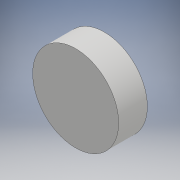
# Autodesk Inventor part: Spacer
Saved by Autodesk Inventor 2017 (Build 210142000, 142)
## iProperties
Created: 2018-02-08
Part Number: Spacer
Material: Generic
Document SubType Name: Modeling
Designer: Arjuna
Density: 1 g/cm^3
Appearance: Default
Author: Arjuna
Autodesk Inventor part; units mm, degrees
ref_plane "YZ Plane" through (0, 0, 0) normal (1, 0, 0) x (0, 1, 0)
ref_plane "XZ Plane" through (0, 0, 0) normal (0, 1, 0) x (-1, 0, 0)
ref_plane "XY Plane" through (0, 0, 0) normal (0, 0, 1) x (1, 0, 0)
sketch "Sketch1" plane through (0, 0, 0) normal (0, 0, 1) x (1, 0, 0)
  line L0 (0, 0) -> (7.5, 0)
  line L1 (7.5, 0) -> (7.5, 5)
  line L2 (7.5, 5) -> (0, 5)
  line L3 (0, 5) -> (0, 0)
  dimension "d0" = 7.5
  dimension "d1" = 5
  constraints: 8 end point, 2 horizontal, 2 perpendicular
  measures "d0" distance of L0.start L0.end
  measures "d1" distance of L0.end L1.end
revolve "Revolution1" add sketch "Sketch1" angle 360 about axis through (0, 5, 0) along (0, -1, 0)
body "Solid1"
